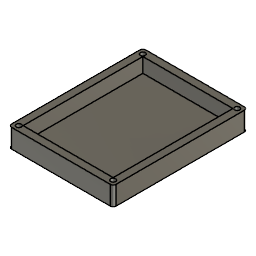
JONAH BASE (Autodesk Fusion 360 design; units mm, degrees)
part number: 2026-01-30-09-33-29-986
Autodesk Fusion 360 part; units mm, degrees
sketch "Sketch1" plane through (0, 0, 0) normal (0, 0, 1) x (1, 0, 0)
  line L0 (0, 0) -> (0, 92.3036)
  line L1 (0, 0) -> (71.9074, 0)
  line L2 (71.9074, 0) -> (71.9074, 92.3036)
  line L3 (71.9074, 92.3036) -> (0, 92.3036)
  line L4 (5, 5) -> (66.9074, 5)
  line L5 (66.9074, 5) -> (66.9074, 87.3036)
  line L6 (66.9074, 87.3036) -> (5, 87.3036)
  line L7 (5, 5) -> (5, 87.3036)
  dimension "d1" = 92.3036
  dimension "d2" = 71.9074
  dimension "d3" = 5
  constraint coincident L0.start L1.start
  constraint vertical L0
  constraint perpendicular L0 L1
  constraint perpendicular L1 L2
  constraint perpendicular L0 L3
  measures "d1" distance of L0.start L0.end
  measures "d2" distance of L0.start L1.end
extrude "Extrude1" add sketch "Sketch1" against normal blind 3 contours L0 L1 L2 L3 | L4 L5 L6 L7
extrude "Extrude2" add sketch "Sketch1" along normal blind 10
fillet "Fillet1" radius 2 4 edges at (71.9074, 0, 3.5) (0, 0, 3.5) (0, 92.3036, 3.5) (71.9074, 92.3036, 3.5)
sketch "Sketch2" plane through (0, 0, 10) normal (0, 0, 1) x (-1, 0, 0)
  line L0 (-66.9074, -87.3036) -> (-66.9074, -5)
  line L1 (-66.9074, -5) -> (-5, -5)
  line L2 (-5, -5) -> (-5, -87.3036)
  line L3 (-5, -87.3036) -> (-66.9074, -87.3036)
  arc A0 (-71.9074, -90.3036) -> (-69.9074, -92.3036) centre (-69.9074, -90.3036) ccw
  line L4 (-69.9074, -92.3036) -> (-2, -92.3036)
  arc A1 (-2, -92.3036) -> (0, -90.3036) centre (-2, -90.3036) ccw
  line L5 (0, -90.3036) -> (0, -2)
  arc A2 (0, -2) -> (-2, 0) centre (-2, -2) ccw
  line L6 (-2, 0) -> (-69.9074, 0)
  arc A3 (-69.9074, 0) -> (-71.9074, -2) centre (-69.9074, -2) ccw
  line L7 (-71.9074, -2) -> (-71.9074, -90.3036)
  circle A4 centre (-68.4022, -3.5052) radius 1.7145
  line L8 (-35.9537, -92.3036) -> (-35.9537, 0)
  circle A5 centre (-3.5052, -3.5052) radius 1.7145
  line L9 (-67.4347, -46.1518) -> (-71.9074, -46.1518)
  line L10 (-67.4347, -46.1518) -> (0, -46.1518)
  circle A6 centre (-68.4022, -88.7984) radius 1.7145
  circle A7 centre (-3.5052, -88.7984) radius 1.7145
  dimension "d12" = 3.429
  constraint midpoint L4 L8.start
  constraint midpoint L6 L8.end
  constraint symmetric A4 L8 A5
  constraint midpoint L7 L9.end
  constraint midpoint L5 L10.end
  constraint perpendicular L5 L10
  constraint symmetric A4 L10 A6
  constraint symmetric A5 L10 A7
  measures "d12" diameter of A4
extrude "Extrude3" cut sketch "Sketch2" against normal blind 5 contours A4 | A5 | A6 | A7
